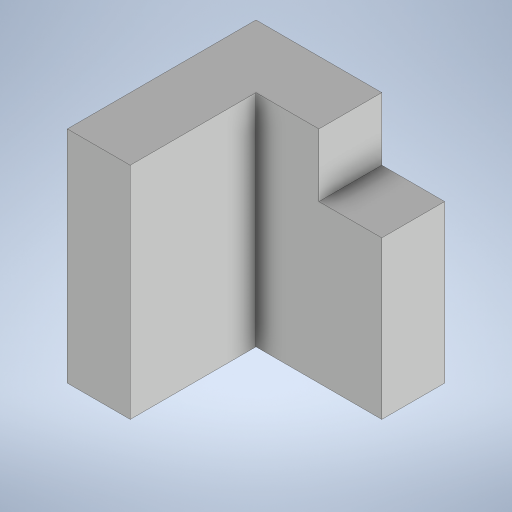
# Autodesk Inventor part: BT001_Winkel
Saved by Autodesk Inventor 2023 (Build 270158000, 158)
## iProperties
Created: 2022-04-24
Part Number: BT001_Winkel
Material: Generic
Document SubType Name: Modeling
Designer: Altar
Density: 1 g/cm^3
Appearance: Default
Author: Altar
Autodesk Inventor part; units mm, degrees
ref_plane "YZ Plane" through (0, 0, 0) normal (1, 0, 0) x (0, 1, 0)
ref_plane "XZ Plane" through (0, 0, 0) normal (0, 1, 0) x (-1, 0, 0)
ref_plane "XY Plane" through (0, 0, 0) normal (0, 0, 1) x (1, 0, 0)
sketch "Sketch1" plane through (0, 0, 0) normal (0, 0, 1) x (1, 0, 0)
  line L0 (-31.9173, -28.8857) -> (-31.9173, 31.1143)
  line L1 (-31.9173, 31.1143) -> (28.0827, 31.1143)
  line L2 (28.0827, 31.1143) -> (28.0827, 11.1143)
  line L3 (28.0827, 11.1143) -> (-11.9173, 11.1143)
  line L4 (-11.9173, 11.1143) -> (-11.9173, -28.8857)
  line L5 (-11.9173, -28.8857) -> (-31.9173, -28.8857)
  point P0 (0, 0)
  dimension "d0" = 60
  dimension "d1" = 20
  dimension "d2" = 60
  dimension "d3" = 20
  constraints: 12 end point, 5 perpendicular, 1 vertical
  measures "d0" distance of L0.end L1.end
  measures "d1" distance of L1.end L2.end
  measures "d2" distance of L0.start L0.end
  measures "d3" distance of L4.end L0.start
extrude "Extrusion1" add sketch "Sketch1" against normal blind 70
sketch "Sketch2" plane through (0, 0, 0) normal (0, 1, 0) x (-1, 0, 0)
  line L0 (-28.0827, 0) -> (31.9173, 0) projected
  line L1 (-28.0827, 0) -> (-8.0827, 0)
  line L2 (-8.0827, 0) -> (-8.0827, -20)
  line L3 (-8.0827, -20) -> (-28.0827, -20)
  line L4 (-28.0827, -20) -> (-28.0827, 0)
  point P0 (0, 0)
  dimension "d6" = 20
  dimension "d7" = 20
  constraints: 8 end point, 3 perpendicular, 1 point on line
  measures "d6" distance of L0.start L1.end
  measures "d7" distance of L1.end L2.end
extrude "Extrusion2" cut sketch "Sketch2" along normal blind 70
body "Solid1"
